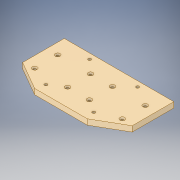
# Autodesk Inventor part: DPLX_P035 Spark Gap Shielding Middle
Saved by Autodesk Inventor 2018 (Build 220112000, 112)
## iProperties
Created: 2017-11-28
Part Number: DPLX_P035 Spark Gap Shielding Middle
Material: Polyethylene, High Density
Document SubType Name: Modeling
Designer: Sam
Density: 0.952 g/cm^3
Appearance: Smooth - Off-White
Mass: 47.182 g
Surface Area: 186.295 cm^2
Volume: 49.5609 cm^3
Author: Sam
Comments: http://www.eplastics.com/Plastic/G9-G10-FR4-glass-epoxy-sheet/G10NAT-250X12X12
Autodesk Inventor part; units mm, degrees
ref_plane "YZ Plane" through (0, 0, 0) normal (1, 0, 0) x (0, 1, 0)
ref_plane "XZ Plane" through (0, 0, 0) normal (0, 1, 0) x (-1, 0, 0)
ref_plane "XY Plane" through (0, 0, 0) normal (0, 0, 1) x (1, 0, 0)
sketch "Sketch1" plane through (0, 0, 0) normal (0, 1, 0) x (-1, 0, 0)
  line L0 (-63.5, 33.655) -> (63.5, 33.655)
  line L1 (63.5, 33.655) -> (63.5, -33.655)
  line L2 (63.5, -33.655) -> (-63.5, -33.655)
  line L3 (-63.5, -33.655) -> (-63.5, 33.655)
  line L4 (-63.5, 33.655) -> (63.5, -33.655) construction
  line L5 (63.5, 33.655) -> (-63.5, -33.655) construction
  point P0 (0, 0)
  dimension "d0" = 127
  dimension "d1" = 67.31
  constraints: 12 end point, 2 midpoint, 2 parallel, 1 horizontal, 1 perpendicular
  measures "d0" distance of L1.end L2.end
  measures "d1" distance of L0.end L1.end
extrude "Extrusion1" add sketch "Sketch1" along normal mid plane 6.35
sketch "Sketch4" plane through (0, 3.175, 0) normal (0, 1, 0) x (1, 0, 0)
  line L0 (63.5, 33.655) -> (-63.5, 33.655) projected
  line L1 (-63.5, -33.655) -> (63.5, -33.655) projected
  line L2 (-63.5, 33.655) -> (-63.5, -33.655) projected
  line L3 (63.5, -33.655) -> (63.5, 33.655) projected
  point P0 (0, 0)
  point P1 (-50.8, 13.335)
  point P2 (-50.8, -13.335)
  point P3 (-12.7, 13.335)
  point P4 (-12.7, -13.335)
  point P5 (12.7, 13.335)
  point P6 (12.7, -13.335)
  point P7 (50.8, 13.335)
  point P8 (50.8, -13.335)
  point P9 (-50.8, -33.655)
  point P10 (50.8, -33.655)
  point P11 (-63.5, -20.955)
  point P12 (63.5, -20.955)
  dimension "d24" = 20.32
  dimension "d25" = 20.32
  dimension "d26" = 12.7
  dimension "d27" = 12.7
  dimension "d28" = 50.8
  dimension "d29" = 50.8
  constraints: 6 horizontal alignment, 4 vertical alignment
  measures "d24" distance from line of L0 point (-50.8, 13.335)
  measures "d25" distance from line of L1 point (-50.8, -13.335)
  measures "d26" distance from line of L2 point (-50.8, 13.335)
  measures "d27" distance from line of point (50.8, 13.335) L3
  measures "d28" distance from line of point (12.7, 13.335) L3
  measures "d29" distance from line of point (-12.7, 13.335) L2
hole "Hole2" at (-50.8, 3.175, -13.335) at (-50.8, 3.175, 13.335) at (-12.7, 3.175, -13.335) at (-12.7, 3.175, 13.335) at (12.7, 3.175, -13.335) at (12.7, 3.175, 13.335) at (50.8, 3.175, -13.335) at (50.8, 3.175, 13.335) direction (0, -1, 0) diameter 3 depth 25.4 tip angle 118 countersink diameter 5.6 countersink angle 90
chamfer "Chamfer1" distance 19.05 angle 60 1 edges at (-63.5, 0, 33.655) measured on face at (-63.5, -1.0583, 11.2183)
sketch "Sketch5" plane through (0, -3.175, 0) normal (0, -1, 0) x (1, 0, 0)
  circle A0 centre (-27.7751, 23.3958) radius 1.7018 projected
  circle A1 centre (27.7749, 23.3958) radius 1.7018 projected
  circle A2 centre (27.7749, -27.4042) radius 1.7018 projected
  circle A3 centre (-27.7751, -27.4042) radius 1.7018 projected
  point P0 (0, 0)
hole "Hole3" at (-27.7751, -3.175, 23.3958) at (27.7749, -3.175, 23.3958) at (27.7749, -3.175, -27.4042) at (-27.7751, -3.175, -27.4042) direction (0, 1, 0) diameter 3.4036 end through all countersink diameter 6.2992 countersink angle 90 clearance for "Flat Head Machine Screw" size "M3" standard "Ansi Metric M Profile"
chamfer "Chamfer2" distance 19.05 angle 60 1 edges at (63.5, 0, 33.655) measured on face at (63.5, 1.0583, 11.2183)
equation "\"d25\" = d24"
equation "\"d27\" = d26"
equation "\"d28\" = d29"
body "Solid1"
